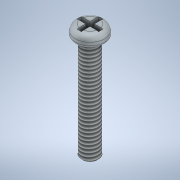
# Autodesk Inventor part: M2_Short_Bolt
Saved by Autodesk Inventor 2021 (Build 250183000, 183)
## iProperties
Created: 2021-09-29
Part Number: M2_Short_Bolt
Material: Generic
Document SubType Name: Modeling
Designer: ermoz
Density: 1 g/cm^3
Appearance: Default
Author: ermoz
Autodesk Inventor part; units mm, degrees
ref_plane "YZ Plane" through (0, 0, 0) normal (1, 0, 0) x (0, 1, 0)
ref_plane "XZ Plane" through (0, 0, 0) normal (0, 1, 0) x (-1, 0, 0)
ref_plane "XY Plane" through (0, 0, 0) normal (0, 0, 1) x (1, 0, 0)
sketch "Sketch1" plane through (0, 0, 0) normal (0, 1, 0) x (-1, 0, 0)
  circle A0 centre (0, 0) radius 1
  dimension "d0" = 2
  constraints: 1 centre point, 1 coincident
  measures "d0" diameter of A0
extrude "Extrusion1" add sketch "Sketch1" along normal blind 13.3
sketch "Sketch2" plane through (0, 13.3, 0) normal (0, 1, 0) x (1, 0, 0)
  circle A0 centre (0, 0) radius 1 projected
  circle A1 centre (0, 0) radius 1.7
  dimension "d3" = 3.4
  constraints: 1 centre point, 1 coincident
  measures "d3" diameter of A1
extrude "Extrusion2" add sketch "Sketch2" against normal blind 1.3 contours A0 | A1
thread "Thread1" size "M2x0.4" class "6g" standard "ANSI Metric M Profile" full length
sketch "Sketch3" plane through (0, 13.3, 0) normal (0, 1, 0) x (1, 0, 0)
  line L0 (-1.25, -0.25) -> (1.25, -0.25)
  line L1 (1.25, -0.25) -> (1.25, 0.25)
  line L2 (1.25, 0.25) -> (-1.25, 0.25)
  line L3 (-1.25, 0.25) -> (-1.25, -0.25)
  line L4 (-1.25, -0.25) -> (1.25, 0.25) construction
  line L5 (1.25, -0.25) -> (-1.25, 0.25) construction
  line L6 (-0.25, 1.25) -> (0.25, 1.25)
  line L7 (0.25, 1.25) -> (0.25, -1.25)
  line L8 (0.25, -1.25) -> (-0.25, -1.25)
  line L9 (-0.25, -1.25) -> (-0.25, 1.25)
  circle A0 centre (0, 0) radius 1 projected
  line L10 (-0.25, 1.25) -> (0.25, -1.25) construction
  line L11 (0.25, 1.25) -> (-0.25, -1.25) construction
  point P0 (-0.25, -0.25)
  point P1 (0.25, -0.25)
  point P2 (0.25, 0.25)
  point P3 (-0.25, 0.25)
  dimension "d8" = 2.5
  dimension "d9" = 0.5
  dimension "d10" = 0.5
  dimension "d11" = 2.5
  constraints: 24 end point, 4 midpoint, 4 parallel, 2 horizontal, 2 perpendicular
  measures "d8" distance of L2.end L1.end
  measures "d9" distance of L1.end L0.end
  measures "d10" distance of L7.end L8.end
  measures "d11" distance of L6.end L7.end
extrude "Extrusion3" cut sketch "Sketch3" against normal blind 1 contours L3 L2 A0 L0 | A0 L2 L9 L0 | L9 L2 L7 L0 | L0 L7 A0 L9 | A0 L7 L8 L9 | L7 L2 A0 L0 | L9 A0 L7 L2 | L9 L6 L7 A0 | A0 L2 L1 L0
chamfer "Chamfer1" distance 0.2 angle 45 1 edges at (1, 0, 0)
fillet "Fillet1" radius 0.65 1 edges at (-1.7, 13.3, 0)
fillet "Fillet2" radius 0.3 1 edges at (-1.7, 12, 0)
body "Solid1"
